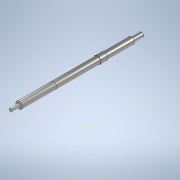
# Autodesk Inventor part: Eje
Saved by Autodesk Inventor 2021 (Build 250183000, 183)
## iProperties
Created: 2020-11-24
Part Number: Eje
Material: Acero, carbono
Document SubType Name: Modeling
Designer: juanm
Density: 7.85 g/cm^3
Appearance: Semipulido
Author: juanm
Autodesk Inventor part; units mm, degrees
ref_plane "YZ Plane" through (0, 0, 0) normal (1, 0, 0) x (0, 1, 0)
ref_plane "XZ Plane" through (0, 0, 0) normal (0, 1, 0) x (-1, 0, 0)
ref_plane "XY Plane" through (0, 0, 0) normal (0, 0, 1) x (1, 0, 0)
sketch "Boceto1" plane through (0, 0, 0) normal (0, 0, 1) x (1, 0, 0)
  circle A0 centre (-235.9106, 152.9734) radius 16.8656
  point P0 (0, 0)
  dimension "d2" = 33.7312
  constraints: 1 centre point
  measures "d2" diameter of A0
extrude "Extrusión1" add sketch "Boceto1" along normal blind 76.2
sketch "Boceto2" plane through (-235.9106, 152.9734, 76.2) normal (0, 0, 1) x (1, 0, 0)
  circle A0 centre (0, 0) radius 24.9682
  point P0 (235.9106, -152.9734)
  dimension "d5" = 49.9364
  constraints: 1 centre point
  measures "d5" diameter of A0
extrude "Extrusión2" add sketch "Boceto2" along normal blind 203.2
sketch "Boceto3" plane through (-235.9106, 152.9734, 279.4) normal (0, 0, 1) x (1, 0, 0)
  circle A0 centre (0, 0) radius 28.0035
  point P0 (235.9106, -152.9734)
  dimension "d8" = 56.007
  constraints: 1 centre point
  measures "d8" diameter of A0
extrude "Extrusión3" add sketch "Boceto3" along normal blind 50.8
sketch "Boceto4" plane through (-235.9106, 152.9734, 330.2) normal (0, 0, 1) x (1, 0, 0)
  circle A0 centre (0, 0) radius 25.654
  point P0 (235.9106, -152.9734)
  dimension "d11" = 51.308
  constraints: 1 centre point
  measures "d11" diameter of A0
extrude "Extrusión4" add sketch "Boceto4" along normal blind 330.2
sketch "Boceto5" plane through (-235.9106, 152.9734, 660.4) normal (0, 0, 1) x (1, 0, 0)
  point P0 (235.9106, -152.9734)
sketch "Boceto6" plane through (-235.9106, 152.9734, 660.4) normal (0, 0, 1) x (1, 0, 0)
  circle A0 centre (0, 0) radius 25.6032
  point P0 (235.9106, -152.9734)
  dimension "d14" = 51.2064
  constraints: 1 centre point
  measures "d14" diameter of A0
extrude "Extrusión5" add sketch "Boceto6" along normal blind 254
sketch "Boceto7" plane through (-235.9106, 152.9734, 914.4) normal (0, 0, 1) x (1, 0, 0)
  circle A0 centre (0, 0) radius 11.6078
  point P0 (235.9106, -152.9734)
  dimension "d17" = 23.2156
  constraints: 1 centre point
  measures "d17" diameter of A0
extrude "Extrusión6" add sketch "Boceto7" along normal blind 63.5
sketch "Boceto8" plane through (-235.9106, 152.9734, 330.2) normal (0, 0, 1) x (1, 0, 0)
  point P0 (235.9106, -152.9734)
sketch "Boceto9" plane through (-235.9106, 152.9734, 977.9) normal (0, 0, 1) x (1, 0, 0)
  point P0 (235.9106, -152.9734)
